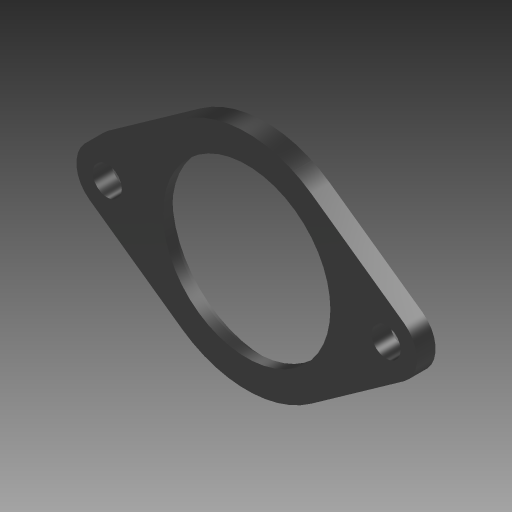
# Autodesk Inventor part: Bearing Retainer
Saved by Autodesk Inventor 2023 (Build 270158000, 158)
## iProperties
Created: 2022-07-04
Part Number: Bearing Retainer
Material: Aluminum 6061
Document SubType Name: Modeling
Designer: Max Boord
Mass: 5.91558 g
Surface Area: 23.905 cm^2
Volume: 2.19095 cm^3
Density: 2.7 g/cm^3
Appearance: Glossy - Black
Mass: 6.49248 g
Surface Area: 26.4386 cm^2
Volume: 2.40462 cm^3
Author: Max Boord
Autodesk Inventor part; units mm, degrees
ref_plane "YZ Plane" through (0, 0, 0) normal (1, 0, 0) x (0, 1, 0)
ref_plane "XZ Plane" through (0, 0, 0) normal (0, 1, 0) x (-1, 0, 0)
ref_plane "XY Plane" through (0, 0, 0) normal (0, 0, 1) x (1, 0, 0)
sketch "Sketch1" plane through (0, 0, 0) normal (0, 0, 1) x (1, 0, 0)
  circle A0 centre (0, 0) radius 15.875
  circle A1 centre (0, 0) radius 19.05
  circle A2 centre (-23.8125, 0) radius 2.4892
  circle A3 centre (-23.8125, 0) radius 5.2705
  line L0 (-26.8624, 4.2984) -> (-11.0236, 15.5365)
  line L1 (-26.8624, -4.2984) -> (-11.0236, -15.5365)
  line L2 (0, 0) -> (0, 8.9484)
  circle A4 centre (23.8125, 0) radius 2.4892
  circle A5 centre (23.8125, 0) radius 5.2705
  line L3 (26.8624, 4.2984) -> (11.0236, 15.5365)
  line L4 (26.8624, -4.2984) -> (11.0236, -15.5365)
  circle A6 centre (0, 0) radius 14.2875
  point P0 (11.0236, -15.5365)
  point P1 (11.0236, 15.5365)
  dimension "d0" = 31.75
  dimension "d1" = 3.175
  dimension "d2" = 4.9784
  dimension "d3" = 10.541
  dimension "d4" = 47.625
  dimension "d5" = 28.575
  constraints: 10 end point, 7 centre point, 6 point on circle, 5 symmetric about line, 4 tangent, 1 coincident, 1 horizontal alignment, 1 vertical, 2 other
  measures "d0" diameter of A0
  measures "d1" radial gap between concentric circles of A0 A1
  measures "d2" diameter of A2
  measures "d3" diameter of A3
  measures "d4" diameter of A2.centre L2
  measures "d5" diameter of A6
extrude "Extrusion1" add sketch "Sketch1" along normal blind 1.5875 contours A0 | A1 A5 A3 | L3 A5 A1 | A1 A3 L0 | A5 A1 | A1 A5 | A3 A1 | A1 A3 | A5 L4 A1 | A1 L1 A3
extrude "Extrusion2" add sketch "Sketch1" against normal blind 1.5875 contours A1 A5 A3 | L3 A5 A1 | A1 A3 L0 | A5 A1 | A1 A5 | A3 A1 | A1 A3 | A5 L4 A1 | A1 L1 A3
body "Solid1"
